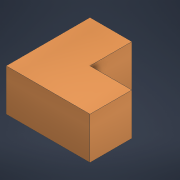
# Autodesk Inventor part: 110033226_ipt_31_城堡四圓塔的頂部角落
Saved by Autodesk Inventor 2022 (Build 260153000, 153)
## iProperties
Created: 2022-06-24
Part Number: 110033226_ipt_31_城堡四圓塔的頂部角落
Material: 一般
Document SubType Name: Modeling
Designer: User
Density: 1 g/cm^3
Appearance: 預設
Author: User
Autodesk Inventor part; units mm, degrees
ref_plane "YZ Plane" through (0, 0, 0) normal (1, 0, 0) x (0, 1, 0)
ref_plane "XZ Plane" through (0, 0, 0) normal (0, 1, 0) x (-1, 0, 0)
ref_plane "XY Plane" through (0, 0, 0) normal (0, 0, 1) x (1, 0, 0)
sketch "草圖1" plane through (0, 0, 0) normal (0, 1, 0) x (-1, 0, 0)
  line L0 (0, 0) -> (0, -5)
  line L1 (0, -5) -> (5, -5)
  line L2 (5, -5) -> (5, -10)
  line L3 (5, -10) -> (10, -10)
  line L4 (10, -10) -> (10, 0)
  line L5 (10, 0) -> (0, 0)
  circle A0 centre (7.5, -2.5) radius 1.7
  line L6 (10, -15) -> (10, -5)
  circle A1 centre (7.5, -7.5) radius 1.7
  line L7 (5, -10) -> (5, 0)
  circle A2 centre (2.5, -2.5) radius 1.7
  line L8 (5, -15) -> (5, -5)
  circle A3 centre (2.5, -7.5) radius 1.7
  dimension "d0" = 10
  dimension "d1" = 5
  dimension "d2" = 5
  dimension "d3" = 5
  dimension "d4" = 3.4
  dimension "d5" = 2.5
  dimension "d6" = 2.5
  dimension "d9" = 5
  dimension "d12" = 5
  constraints: 18 end point, 5 perpendicular, 4 centre point, 2 vertical, 1 horizontal, 15 other
  measures "d0" distance of L3.end L4.end
  measures "d1" distance of L0.start L0.end
  measures "d2" distance of L0.end L1.end
  measures "d3" distance of L2.end L3.end
  measures "d4" diameter of A0
  measures "d5" distance from line of L4 A0.centre
  measures "d6" distance from line of L5 A0.centre
  measures "d9" distance of L3.end L6.start
  measures "d12" distance of L3.end L7.start
extrude "擠出1" add sketch "草圖1" along normal blind 5 contours L5 L7 L1 L0 | L5 L4 L3 L2 L7 | A0 | A1 | A2
sketch "草圖2" plane through (0, 0, 0) normal (0, -1, 0) x (1, 0, 0)
  circle A0 centre (-2.5, -2.5) radius 1.7 projected
  circle A1 centre (-7.5, -2.5) radius 1.7 projected
  circle A2 centre (-7.5, -7.5) radius 1.7 projected
  point P0 (0, 0)
extrude "擠出2" cut sketch "草圖2" against normal blind 1.5
